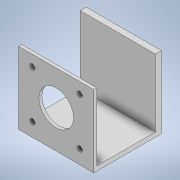
# Autodesk Inventor part: Motorhalterung_v2
Saved by Autodesk Inventor 2021 (Build 250183000, 183)
## iProperties
Created: 2021-01-03
Part Number: Motorhalterung_v2
Material: Generisch
Document SubType Name: Modeling
Designer: Ctroi
Density: 1 g/cm^3
Appearance: Vorgabe
Author: Ctroi
## iProperties of the stored document _3D-Druck.ipt
Created: 2021-01-04
Part Number: _3D-Druck
Material: Generisch
Document SubType Name: Modeling
Designer: Ctroi
Density: 1 g/cm^3
Appearance: Vorgabe
Author: Ctroi
Autodesk Inventor part; units mm, degrees
ref_plane "YZ Plane" through (0, 0, 0) normal (1, 0, 0) x (0, 1, 0)
ref_plane "XZ Plane" through (0, 0, 0) normal (0, 1, 0) x (-1, 0, 0)
ref_plane "XY Plane" through (0, 0, 0) normal (0, 0, 1) x (1, 0, 0)
sketch "Skizze1" plane through (0, 0, 0) normal (0, 1, 0) x (-1, 0, 0)
  line L0 (-25, 22.5) -> (25, 22.5)
  line L1 (25, 22.5) -> (25, -22.5)
  line L2 (25, -22.5) -> (-25, -22.5)
  line L3 (-25, -22.5) -> (-25, 22.5)
  line L4 (0, -31.5) -> (0, 31.5) projected
  line L5 (35, 0) -> (-35, 0) projected
  point P0 (0, 0)
  dimension "d0" = 50
  dimension "d1" = 45
  constraints: 8 end point, 2 parallel, 1 horizontal, 1 perpendicular, 2 other
  measures "d0" distance of L1.end L2.end
  measures "d1" distance of L0.end L1.end
extrude "Extrusion1" add sketch "Skizze1" along normal blind 3
sketch "Skizze2" plane through (0, 3, 0) normal (0, 1, 0) x (1, 0, 0)
  line L0 (-25, 22.5) -> (-25, -22.5) projected
  line L1 (25, -22.5) -> (25, 22.5) projected
  line L2 (-25, -22.5) -> (25, -22.5)
  line L3 (25, -22.5) -> (25, -20.5)
  line L4 (25, -20.5) -> (-25, -20.5)
  line L5 (-25, -20.5) -> (-25, -22.5)
  point P0 (0, 0)
  point P1 (-25, -20.5)
  dimension "d4" = 2
  constraints: 8 end point, 2 parallel, 1 horizontal, 1 perpendicular, 1 point on line
  measures "d4" distance of L3.end L2.end
extrude "Extrusion2" add sketch "Skizze2" along normal blind 45
sketch "Skizze3" plane through (-25, 0, 22.5) normal (0, 0, 1) x (1, 0, 0)
  circle A0 centre (25, 25) radius 11.5
  line L0 (0, 0) -> (50, 0) projected
  line L1 (50, 0) -> (50, 48) projected
  circle A1 centre (40.75, 9.25) radius 1.75
  circle A2 centre (9.25, 9.25) radius 1.75
  circle A3 centre (9.25, 40.75) radius 1.75
  circle A4 centre (40.75, 40.75) radius 1.75
  line L2 (0, 48) -> (50, 48) projected
  line L3 (25, 48) -> (25, 0)
  line L4 (-0.3792, 25) -> (50, 25)
  dimension "d7" = 23
  dimension "d8" = 25
  dimension "d10" = 3.5
  dimension "d11" = 3.5
  dimension "d12" = 3.5
  dimension "d13" = 3.5
  dimension "d17" = 31.5
  constraints: 5 centre point, 4 end point, 3 symmetric about line, 2 perpendicular, 1 midpoint, 1 point on line
  measures "d7" diameter of A0
  measures "d8" distance from line of L0 A0.centre
  measures "d10" diameter of A1
  measures "d11" diameter of A2
  measures "d12" diameter of A3
  measures "d13" diameter of A4
  measures "d17" diameter of A4.centre L3
extrude "Extrusion3" cut sketch "Skizze3" against normal up to surface (2 mm away) contours L4 L3 A0 | A0 L3 L4 | L3 L4 A0 | A0 L4 L3 | A1 | A2 | A3 | A4
sketch "Skizze6" plane through (0, 3, 0) normal (0, 1, 0) x (1, 0, 0)
  line L0 (25, 22.5) -> (-25, 22.5) projected
  line L1 (-25, 22.5) -> (25, 22.5)
  line L2 (25, 22.5) -> (25, 18.5)
  line L3 (25, 18.5) -> (-25, 18.5)
  line L4 (-25, 18.5) -> (-25, 22.5)
  point P0 (0, 0)
  dimension "d25" = 50
  dimension "d26" = 4
  constraints: 8 end point, 2 parallel, 1 horizontal, 1 perpendicular
  measures "d25" distance of L2.end L3.end
  measures "d26" distance of L1.end L2.end
extrude "Extrusion5" add sketch "Skizze6" along normal blind 45
